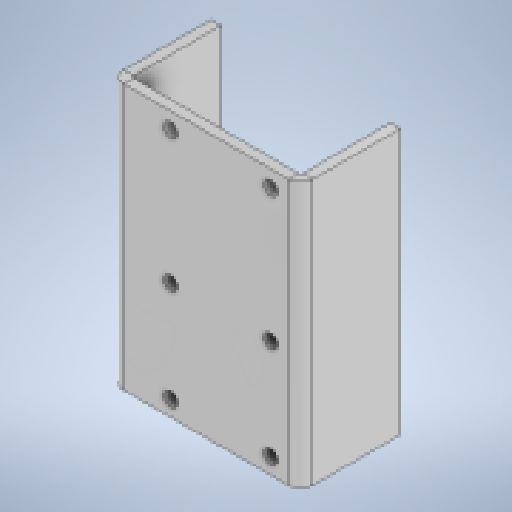
# Autodesk Inventor part: body_motor_L_frame
Saved by Autodesk Inventor 2025.2 (Build 292293000, 293)
## iProperties
Created: 2025-05-30
Part Number: body_motor_L_frame
Material: Aluminum 6061-AHC
Document SubType Name: Sheet Metal
Designer: chris
Density: 2.7 g/cm^3
Sheet Metal Rule: Default_mm
Appearance: Aluminum - Dark
Author: chris
Autodesk Inventor part; units mm, degrees
ref_plane "YZ Plane" through (0, 0, 0) normal (1, 0, 0) x (0, 1, 0)
ref_plane "XZ Plane" through (0, 0, 0) normal (0, 1, 0) x (-1, 0, 0)
ref_plane "XY Plane" through (0, 0, 0) normal (0, 0, 1) x (1, 0, 0)
sketch "Sketch1" plane through (0, 0, 0) normal (0, 0, 1) x (1, 0, 0)
  line L0 (-14.25, -20) -> (14.25, -20)
  line L1 (14.25, -20) -> (14.25, 20)
  line L2 (14.25, 20) -> (-14.25, 20)
  line L3 (-14.25, 20) -> (-14.25, -20)
  line L4 (-14.25, -20) -> (14.25, 20) construction
  line L5 (14.25, -20) -> (-14.25, 20) construction
  point P0 (0, 0)
  dimension "d0" = 28.5
  dimension "d1" = 40
  measures "d0" distance of L1.end L2.end
  measures "d1" distance of L0.end L1.end
extrude "Plate1" add sketch "Sketch1" along normal blind 1.5
sketch "Sketch2" plane through (12.75, -20, 1.5) normal (1, 0, 0) x (0, 1, 0)
  line L0 (40, 0) -> (0, 0)
  line L1 (0, 0) -> (0, -15)
  line L2 (0, -15) -> (40, -15)
  line L3 (40, -15) -> (40, 0)
  constraints: 6 end point, 1 horizontal, 1 perpendicular, 1 vertical
edge flange "Flange1" height 15 angle 90 thickness 1.5 bend radius 0.31 thickness toward (1, 0, 0) relief straight relief width 1.5 relief depth 0.75 corner gap 0.31 corner form 0 edges at (14.25, 0, 0) (-14.25, 0, 0) wall of the first edge with corners at (12.75, 20, 1.5) (12.75, -20, 1.5) (12.75, -20, -13.5) (12.75, 20, -13.5)
bend "Bend1"
corner "Corner1"
sketch "Sketch3" plane through (0, 0, 1.5) normal (0, 0, 1) x (1, 0, 0)
  ellipse E0 centre (-5.772, 17.882) end of major axis (-6.638, 18.748) minor radius 1 (-5.9956, 19) -> (-6.89, 18.1056) ccw projected
  line L0 (10.3556, 19) -> (-5.9956, 19) projected
  ellipse E1 centre (10.132, 17.882) end of major axis (10.998, 18.748) minor radius 1 (11.25, 18.1056) -> (10.3556, 19) ccw projected
  line L1 (11.25, -18.2056) -> (11.25, 18.1056) projected
  ellipse E2 centre (10.132, -17.982) end of major axis (10.998, -18.848) minor radius 1 (10.3556, -19.1) -> (11.25, -18.2056) ccw projected
  line L2 (-5.9956, -19.1) -> (10.3556, -19.1) projected
  ellipse E3 centre (-5.772, -17.982) end of major axis (-6.638, -18.848) minor radius 1 (-6.89, -18.2056) -> (-5.9956, -19.1) ccw projected
  line L3 (-6.89, 18.1056) -> (-6.89, -18.2056) projected
  circle A0 centre (9.705, -17.6) radius 0.7835 projected
  circle A1 centre (-5.345, -17.6) radius 0.7835 projected
  circle A2 centre (9.705, -2.5) radius 0.7835 projected
  circle A3 centre (-5.345, -2.5) radius 0.7835 projected
  circle A4 centre (9.705, 17.5) radius 0.7835 projected
  circle A5 centre (-5.345, 17.5) radius 0.7835 projected
  circle A6 centre (2.18, 10) radius 6.4 projected
  point P0 (0, 0)
  constraints: 4 other
hole "Hole1" at (-5.345, -17.6, 1.5) at (9.705, -17.6, 1.5) at (9.705, -2.5, 1.5) at (-5.345, -2.5, 1.5) at (-5.345, 17.5, 1.5) at (9.705, 17.5, 1.5) direction (0, 0, -1) diameter 2.1 depth 1.5
sketch "Sketch4" plane through (0, 0, 1.5) normal (0, 0, 1) x (1, 0, 0)
  ellipse E0 centre (-5.772, 17.882) end of major axis (-6.638, 18.748) minor radius 1 (-5.9956, 19) -> (-6.89, 18.1056) ccw projected
  line L0 (10.3556, 19) -> (-5.9956, 19) projected
  ellipse E1 centre (10.132, 17.882) end of major axis (10.998, 18.748) minor radius 1 (11.25, 18.1056) -> (10.3556, 19) ccw projected
  line L1 (11.25, -18.2056) -> (11.25, 18.1056) projected
  ellipse E2 centre (10.132, -17.982) end of major axis (10.998, -18.848) minor radius 1 (10.3556, -19.1) -> (11.25, -18.2056) ccw projected
  line L2 (-5.9956, -19.1) -> (10.3556, -19.1) projected
  ellipse E3 centre (-5.772, -17.982) end of major axis (-6.638, -18.848) minor radius 1 (-6.89, -18.2056) -> (-5.9956, -19.1) ccw projected
  line L3 (-6.89, 18.1056) -> (-6.89, -18.2056) projected
  circle A0 centre (9.705, -17.6) radius 0.7835 projected
  circle A1 centre (-5.345, -17.6) radius 0.7835 projected
  circle A2 centre (9.705, -2.5) radius 0.7835 projected
  circle A3 centre (-5.345, -2.5) radius 0.7835 projected
  circle A4 centre (9.705, 17.5) radius 0.7835 projected
  circle A5 centre (-5.345, 17.5) radius 0.7835 projected
  circle A6 centre (2.18, 10) radius 6.4 projected
  point P0 (0, 0)
  constraints: 4 other
extrude "Extrusion1" cut sketch "Sketch4" against normal blind 1.5 contours A6
equation "\"d18\" = Thickness"
equation "\"d2\" = Thickness"
equation "\"d3\" = BendReliefWidth"
equation "\"d4\" = BendReliefDepth"
equation "\"d5\" = MinimumRemnant"
equation "\"d6\" = TransitionRadius"
equation "\"d9\" = BendRadius"
equation "\"d10\" = CornerReliefSize"
equation "\"d11\" = GapSize"
equation "\"d12\" = JacobiRadiusSize"
equation "\"BendReliefWidth\" = Thickness"
equation "\"BendReliefDepth\" = 0.5 * Thickness"
equation "\"CornerReliefSize\" = 4 * Thickness"
equation "\"MinimumRemnant\" = 2 * Thickness"
equation "\"TransitionRadius\" = BendRadius"
equation "\"JacobiRadiusSize\" = BendRadius"
equation "\"GapSize\" = Thickness"
equation "\"Thickness\" = 1.5"
equation "\"BendRadius\" = 0.31"
body "Solid1"
